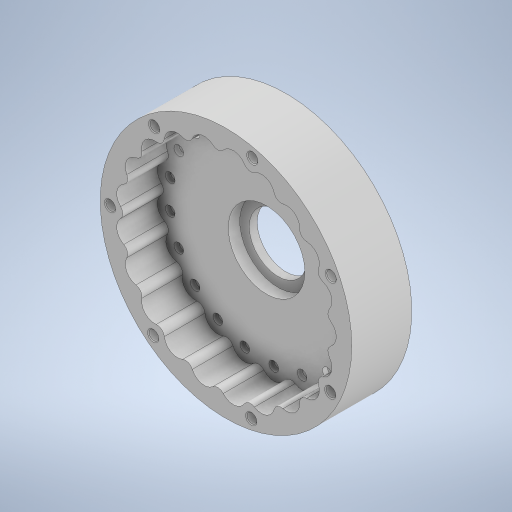
# Autodesk Inventor part: Case
Saved by Autodesk Inventor 2023 (Build 270158000, 158)
## iProperties
Created: 2023-01-17
Part Number: Case
Material: Generic
Document SubType Name: Modeling
Designer: caden
Density: 1 g/cm^3
Appearance: Default
Author: caden
Autodesk Inventor part; units mm, degrees
ref_plane "YZ Plane" through (0, 0, 0) normal (1, 0, 0) x (0, 1, 0)
ref_plane "XZ Plane" through (0, 0, 0) normal (0, 1, 0) x (-1, 0, 0)
ref_plane "XY Plane" through (0, 0, 0) normal (0, 0, 1) x (1, 0, 0)
sketch "Sketch2" plane through (0, 0, 0) normal (0, 0, 1) x (1, 0, 0)
  circle A0 centre (0, 0) radius 77.5
  arc A1 (-64.8986, -3.1989) -> (-64.8986, 3.1989) centre (-68, 0) ccw
  circle A2 centre (-59.3298, -8.9425) radius 3 construction
  circle A3 centre (-59.3298, -8.9425) radius 6.5 construction
  arc A4 (-64.8986, -3.1989) -> (-66.2422, -12.9698) centre (-59.3298, -8.9425) ccw
  line L0 (0, 0) -> (-75.7061, 0) construction
  circle A5 centre (-59.3298, 8.9425) radius 3 construction
  circle A6 centre (-59.3298, 8.9425) radius 6.5 construction
  arc A7 (-66.2422, 12.9698) -> (-64.8986, 3.1989) centre (-59.3298, 8.9425) ccw
  arc A8 (-67.1222, -7.1317) -> (-62.9582, -16.0724) centre (-59.3298, -8.9425) ccw
  arc A9 (-61.0724, -22.186) -> (-62.9582, -16.0724) centre (-64.979, -20.0434) ccw
  arc A10 (-61.0724, -22.186) -> (-59.4764, -31.9188) centre (-54.0581, -26.033) ccw
  arc A11 (-62.0381, -26.5994) -> (-55.4237, -33.9156) centre (-54.0581, -26.033) ccw
  arc A12 (-51.8197, -39.2017) -> (-55.4237, -33.9156) centre (-56.1842, -38.3058) ccw
  arc A13 (-51.8197, -39.2017) -> (-47.4258, -48.0317) centre (-43.9831, -40.8104) ccw
  arc A14 (-51.4416, -43.7037) -> (-42.9646, -48.7453) centre (-43.9831, -40.8104) ccw
  arc A15 (-37.9626, -52.7342) -> (-42.9646, -48.7453) centre (-42.3973, -53.1645) ccw
  arc A16 (-37.9626, -52.7342) -> (-31.1612, -59.8768) centre (-30, -51.9615) ccw
  arc A17 (-36.2743, -56.9248) -> (-26.6879, -59.2437) centre (-30, -51.9615) ccw
  arc A18 (-20.7323, -61.581) -> (-26.6879, -59.2437) centre (-24.8432, -63.2994) ccw
  arc A19 (-20.7323, -61.581) -> (-12.1278, -66.4016) centre (-13.3513, -58.4957) ccw
  arc A20 (-17.8838, -65.0878) -> (-8.0398, -64.478) centre (-13.3513, -58.4957) ccw
  arc A21 (-1.6599, -64.9561) -> (-8.0398, -64.478) centre (-5.0816, -67.8099) ccw
  arc A22 (-1.6599, -64.9561) -> (7.9832, -67.0262) centre (4.4838, -59.8322) ccw
  arc A23 (2.0957, -67.4675) -> (11.3226, -63.9832) centre (4.4838, -59.8322) ccw
  arc A24 (17.56, -62.5596) -> (11.3226, -63.9832) centre (15.1314, -66.2951) ccw
  arc A25 (17.56, -62.5596) -> (27.3849, -61.6954) centre (21.9205, -55.8524) ccw
  arc A26 (21.8889, -63.8524) -> (29.679, -57.8032) centre (21.9205, -55.8524) ccw
  arc A27 (35.2196, -54.6044) -> (29.679, -57.8032) centre (34, -58.8897) ccw
  arc A28 (35.2196, -54.6044) -> (44.3533, -50.8826) centre (37.4094, -46.9099) ccw
  arc A29 (39.7373, -54.5637) -> (45.3982, -46.4872) centre (37.4094, -46.9099) ccw
  arc A30 (49.7498, -41.7973) -> (45.3982, -46.4872) centre (49.8475, -46.2517) ccw
  arc A31 (49.7498, -41.7973) -> (57.3807, -35.5486) centre (49.5743, -33.7992) ccw
  arc A32 (54.0548, -40.4268) -> (57.0836, -31.0405) centre (49.5743, -33.7992) ccw
  arc A33 (59.8595, -25.2763) -> (57.0836, -31.0405) centre (61.2659, -29.5041) ccw
  arc A34 (59.8595, -25.2763) -> (65.3096, -17.056) centre (57.3344, -17.6853) ccw
  arc A35 (63.5693, -22.6978) -> (63.6969, -12.8358) centre (57.3344, -17.6853) ccw
  arc A36 (64.6505, -6.5095) -> (63.6969, -12.8358) centre (67.2405, -10.1349) ccw
  arc A37 (64.6505, -6.5095) -> (67.4354, 2.952) centre (60, 0) ccw
  arc A38 (67.4354, -2.952) -> (64.6505, 6.5095) centre (60, 0) ccw
  arc A39 (63.6969, 12.8358) -> (64.6505, 6.5095) centre (67.2405, 10.1349) ccw
  arc A40 (63.6969, 12.8358) -> (63.5693, 22.6978) centre (57.3344, 17.6853) ccw
  arc A41 (65.3096, 17.056) -> (59.8595, 25.2763) centre (57.3344, 17.6853) ccw
  arc A42 (57.0836, 31.0405) -> (59.8595, 25.2763) centre (61.2659, 29.5041) ccw
  arc A43 (57.0836, 31.0405) -> (54.0548, 40.4268) centre (49.5743, 33.7992) ccw
  arc A44 (57.3807, 35.5486) -> (49.7498, 41.7973) centre (49.5743, 33.7992) ccw
  arc A45 (45.3982, 46.4872) -> (49.7498, 41.7973) centre (49.8475, 46.2517) ccw
  arc A46 (45.3982, 46.4872) -> (39.7373, 54.5637) centre (37.4094, 46.9099) ccw
  arc A47 (44.3533, 50.8826) -> (35.2196, 54.6044) centre (37.4094, 46.9099) ccw
  arc A48 (29.679, 57.8032) -> (35.2196, 54.6044) centre (34, 58.8897) ccw
  arc A49 (29.679, 57.8032) -> (21.8889, 63.8524) centre (21.9205, 55.8524) ccw
  arc A50 (27.3849, 61.6954) -> (17.56, 62.5596) centre (21.9205, 55.8524) ccw
  arc A51 (11.3226, 63.9832) -> (17.56, 62.5596) centre (15.1314, 66.2951) ccw
  arc A52 (11.3226, 63.9832) -> (2.0957, 67.4675) centre (4.4838, 59.8322) ccw
  arc A53 (7.9832, 67.0262) -> (-1.6599, 64.9561) centre (4.4838, 59.8322) ccw
  arc A54 (-8.0398, 64.478) -> (-1.6599, 64.9561) centre (-5.0816, 67.8099) ccw
  arc A55 (-8.0398, 64.478) -> (-17.8838, 65.0878) centre (-13.3513, 58.4957) ccw
  arc A56 (-12.1278, 66.4016) -> (-20.7323, 61.581) centre (-13.3513, 58.4957) ccw
  arc A57 (-26.6879, 59.2437) -> (-20.7323, 61.581) centre (-24.8432, 63.2994) ccw
  arc A58 (-26.6879, 59.2437) -> (-36.2743, 56.9248) centre (-30, 51.9615) ccw
  arc A59 (-31.1612, 59.8768) -> (-37.9626, 52.7342) centre (-30, 51.9615) ccw
  arc A60 (-42.9646, 48.7453) -> (-37.9626, 52.7342) centre (-42.3973, 53.1645) ccw
  arc A61 (-42.9646, 48.7453) -> (-51.4416, 43.7037) centre (-43.9831, 40.8104) ccw
  arc A62 (-47.4258, 48.0317) -> (-51.8197, 39.2017) centre (-43.9831, 40.8104) ccw
  arc A63 (-55.4237, 33.9156) -> (-51.8197, 39.2017) centre (-56.1842, 38.3058) ccw
  arc A64 (-55.4237, 33.9156) -> (-62.0381, 26.5994) centre (-54.0581, 26.033) ccw
  arc A65 (-59.4764, 31.9188) -> (-61.0724, 22.186) centre (-54.0581, 26.033) ccw
  arc A66 (-62.9582, 16.0724) -> (-61.0724, 22.186) centre (-64.979, 20.0434) ccw
  arc A67 (-62.9582, 16.0724) -> (-67.1222, 7.1317) centre (-59.3298, 8.9425) ccw
  point P0 (-62.0381, 26.5994)
  point P1 (-36.2743, 56.9248)
  point P2 (2.0957, 67.4675)
  point P3 (39.7373, 54.5637)
  point P4 (63.5693, 22.6978)
  point P5 (67.4354, 2.952)
  point P6 (57.3807, -35.5486)
  point P7 (7.9832, -67.0262)
  point P8 (-12.1278, -66.4016)
  point P9 (-31.1612, -59.8768)
  point P10 (-47.4258, -48.0317)
  point P11 (-59.4764, -31.9188)
  dimension "d0" = 155
  dimension "d3" = 1.5
  dimension "d4" = 68
  dimension "d7" = 360
  constraints: 126 point on circle, 64 centre point, 4 coincident, 2 end point, 2 tangent, 1 horizontal, 1 point on line, 211 other
  measures "d0" diameter of A0
  measures "d3" radial gap between concentric circles of A4 A3
  measures "d4" distance of point (0, 0) A1.centre
extrude "Extrusion1" add sketch "Sketch2" along normal blind 25
sketch "Sketch3" plane through (0, 0, 0) normal (0, 0, -1) x (-1, 0, 0)
  circle A0 centre (0, 0) radius 77.5
  circle A1 centre (0, 0) radius 77.5 projected
  constraints: 1 centre point, 1 coincident, 1 concentric
extrude "Extrusion2" add sketch "Sketch3" along normal blind 12
sketch "Sketch5" plane through (0, 0, 0) normal (0, 0, 1) x (1, 0, 0)
  point P0 (0, 0)
  point P1 (0, 0)
  constraints: 1 coincident
hole "Hole1" at (0, 0, 0) direction (0, 0, -1) diameter 35.56 end through all counterbore diameter 47.244 counterbore depth 7.112
sketch "Sketch6" plane through (0, 0, 0) normal (0, 0, 1) x (1, 0, 0)
  circle A0 centre (60, 0) radius 3
  arc A1 (64.6505, -6.5095) -> (64.6505, 6.5095) centre (60, 0) ccw projected
  point P0 (0, 0)
  dimension "d23" = 6
  constraints: 1 centre point, 1 coincident
  measures "d23" diameter of A0
extrude "Extrusion4" cut sketch "Sketch6" against normal blind 3
pattern_circular "Circular Pattern1" count 21 over 360 about axis through (0, 0, -3.556) along (0, 0, 1) of "Extrusion4"
sketch "Sketch7" plane through (0, 0, 25) normal (0, 0, 1) x (1, 0, 0)
  circle A0 centre (0, 0) radius 71.5 construction
  point P0 (-71.4991, 0.3515)
  dimension "d39" = 143
  constraints: 1 coincident, 3 other
hole "Hole2" at (-71.4991, 0.3515, 25) direction (0, 0, -1) diameter 6 depth 6 countersink diameter 7 countersink angle 90
pattern_circular "Circular Pattern2" count 7 over 360 about axis through (0, 0, -10) along (0, 0, 1) of "Hole2"
body "Solid1"
